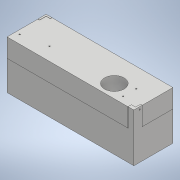
# Autodesk Inventor part: 10руб
Saved by Autodesk Inventor 2020 (Build 240168000, 168)
## iProperties
Created: 2020-02-01
Part Number: 10руб
Material: Типовые
Document SubType Name: Modeling
Designer: Css38
Density: 1 g/cm^3
Appearance: По умолчанию
Author: Css38
Autodesk Inventor part; units mm, degrees
ref_plane "YZ Plane" through (0, 0, 0) normal (1, 0, 0) x (0, 1, 0)
ref_plane "XZ Plane" through (0, 0, 0) normal (0, 1, 0) x (-1, 0, 0)
sketch "Эскиз1" plane through (0, 0, 0) normal (0, 0, 1) x (1, 0, 0)
  line L0 (-76.25, 23.5) -> (76.25, 23.5)
  line L1 (76.25, 23.5) -> (76.25, -23.5)
  line L2 (76.25, -23.5) -> (-76.25, -23.5)
  line L3 (-76.25, -23.5) -> (-76.25, 23.5)
  line L4 (-76.25, 23.5) -> (76.25, -23.5) construction
  line L5 (76.25, 23.5) -> (-76.25, -23.5) construction
  point P0 (0, 0)
  point P1 (0, 0)
  dimension "d35" = 152.5
  dimension "d36" = 47
  constraints: 12 end point, 2 parallel, 1 coincident, 1 horizontal, 1 midpoint, 1 perpendicular
  measures "d35" distance of L1.end L2.end
  measures "d36" distance of L2.end L0.start
extrude "Выдавливание1" add sketch "Эскиз1" along normal blind 30
sketch "Эскиз2" plane through (0, 0, 30) normal (0, 0, 1) x (1, 0, 0)
  line L0 (76.25, 23.5) -> (76.25, -23.5) construction
  line L1 (76.25, -23.5) -> (-76.25, -23.5) construction
  line L2 (-76.25, -23.5) -> (-76.25, 23.5) construction
  line L3 (-76.25, 23.5) -> (76.25, 23.5) construction
  line L4 (74.25, -19.5) -> (50.25, -19.5)
  line L5 (50.25, -19.5) -> (50.25, 4.5)
  line L6 (50.25, 4.5) -> (74.25, 4.5)
  line L7 (74.25, 4.5) -> (74.25, -19.5)
  point P0 (0, 0)
  dimension "d40" = 24
  dimension "d138" = 2
  dimension "d139" = 4
  constraints: 8 end point, 2 parallel, 2 perpendicular, 1 horizontal
  measures "d40" distance of L5.end L6.end
  measures "d138" distance between parallel lines of L0 L7
  measures "d139" distance between parallel lines of L1 L4
extrude "Выдавливание2" cut sketch "Эскиз2" against normal up to next
sketch "Эскиз3" plane through (0, 0, 30) normal (0, 0, 1) x (1, 0, 0)
  line L0 (50.25, 4.5) -> (50.25, -19.5)
  line L1 (50.25, -19.5) -> (74.25, -19.5)
  line L2 (74.25, -19.5) -> (74.25, 4.5)
  line L3 (74.25, 4.5) -> (50.25, 4.5)
  line L4 (76.25, 23.5) -> (76.25, -23.5) construction
  line L5 (76.25, -23.5) -> (-76.25, -23.5) construction
  line L6 (-76.25, 23.5) -> (76.25, 23.5) construction
  line L7 (76.25, 23.5) -> (-76.25, 23.5) projected
  line L8 (-76.25, 23.5) -> (76.25, 23.5)
  line L9 (76.25, 23.5) -> (76.25, -23.5)
  line L10 (76.25, -23.5) -> (-76.25, -23.5)
  line L11 (-76.25, 23.5) -> (-76.25, 21.5)
  line L12 (-76.25, 23.5) -> (-76.25, -23.5) construction
  line L13 (-76.25, 21.5) -> (3.25, 21.5)
  line L14 (3.25, 21.5) -> (3.25, 4.5)
  line L15 (3.25, 4.5) -> (23.25, 4.5)
  line L16 (23.25, 4.5) -> (23.25, -19.5)
  line L17 (23.25, -19.5) -> (-76.25, -19.5)
  line L18 (-76.25, -23.5) -> (-76.25, -19.5)
  line L19 (-76.25, -23.5) -> (76.25, -23.5) projected
  line L20 (76.25, -23.5) -> (76.25, 23.5) projected
  line L21 (74.25, -19.5) -> (50.25, -19.5) projected
  line L22 (50.25, -19.5) -> (50.25, 4.5) projected
  line L23 (50.25, 4.5) -> (74.25, 4.5) projected
  line L24 (74.25, 4.5) -> (74.25, -19.5) projected
  dimension "d50" = 2
  dimension "d52" = 20
  dimension "d63" = 27
  constraints: 34 end point, 13 collinear, 4 perpendicular, 2 parallel, 2 point on line
  measures "d50" distance of L6.start L11.end
  measures "d52" distance between parallel lines of L14 L16
  measures "d63" distance between parallel lines of L0 L16
extrude "Выдавливание4" add sketch "Эскиз3" along normal blind 3
sketch "Эскиз4" plane through (0, 0, 33) normal (0, 0, 1) x (1, 0, 0)
  line L0 (50.25, 4.5) -> (50.25, -19.5) construction
  line L1 (50.25, -19.5) -> (74.25, -19.5) construction
  line L2 (74.25, -19.5) -> (74.25, 4.5) construction
  line L3 (74.25, 4.5) -> (50.25, 4.5) construction
  line L4 (76.25, 23.5) -> (76.25, -23.5) projected
  line L5 (76.25, -23.5) -> (-76.25, -23.5) projected
  line L6 (-76.25, -23.5) -> (-76.25, -19.5) projected
  line L7 (-76.25, -19.5) -> (23.25, -19.5) projected
  line L8 (23.25, -19.5) -> (23.25, 4.5) projected
  line L9 (23.25, 4.5) -> (3.25, 4.5) projected
  line L10 (3.25, 4.5) -> (3.25, 21.5) projected
  line L11 (3.25, 21.5) -> (-76.25, 21.5) projected
  line L12 (-76.25, 21.5) -> (-76.25, 23.5) projected
  line L13 (-76.25, 23.5) -> (76.25, 23.5) projected
  line L14 (23.25, -19.5) -> (23.25, 4.5) projected
  line L15 (23.25, 4.5) -> (50.25, 4.5) construction
  line L16 (50.25, 4.5) -> (50.25, -19.5) projected
  line L17 (50.25, -19.5) -> (23.25, -19.5) construction
  circle A0 centre (36.75, -7.5) radius 11.75
  line L18 (36.75, -7.5) -> (36.75, 4.5) construction
  line L19 (36.75, -7.5) -> (36.75, -19.5) construction
  line L20 (50.25, -19.5) -> (50.25, 4.5) construction
  line L21 (36.75, -7.5) -> (23.25, -7.5) construction
  line L22 (36.75, -7.5) -> (50.25, -7.5) construction
  point P0 (0, 0)
  dimension "d55" = 23.5
  constraints: 12 end point, 4 midpoint, 3 perpendicular, 2 collinear, 1 centre point, 1 point on line, 1 other
  measures "d55" diameter of A0
extrude "Выдавливание7" add sketch "Эскиз4" along normal blind 25
sketch "Эскиз6" plane through (23.25, -19.5, 30) normal (-1, 0, 0) x (0, 0, 1)
  line L0 (3, 0.25) -> (3, 23.75) construction
  line L1 (0, 24) -> (28, 24) projected
  line L2 (0, 0) -> (28, 0) projected
  line L3 (3, 24) -> (5.7, 24)
  line L4 (5.7, 24) -> (5.7, 0)
  line L5 (5.7, 0) -> (3, 0)
  line L6 (3, 0) -> (3, 24)
  point P0 (-30, 19.5)
  dimension "d66" = 2.7
  constraints: 8 end point, 2 parallel, 2 point on line, 1 collinear, 1 horizontal, 1 perpendicular
  measures "d66" distance of L4.end L5.end
extrude "Выдавливание8" cut sketch "Эскиз6" against normal up to surface (51 mm away) from surface at 0
sketch "Эскиз7" plane through (0, 0, 58) normal (0, 0, 1) x (1, 0, 0)
  line L0 (76.25, -23.5) -> (-76.25, -23.5) projected
  line L1 (-76.25, 23.5) -> (76.25, 23.5) projected
  line L2 (76.25, -23.5) -> (-76.25, -23.5)
  line L3 (-76.25, -23.5) -> (-76.25, 23.5)
  line L4 (-76.25, 23.5) -> (76.25, 23.5)
  line L5 (76.25, 23.5) -> (76.25, -23.5)
  circle A0 centre (36.75, -7.5) radius 11.75 projected
  point P0 (0, 0)
  constraints: 8 end point, 2 parallel, 1 horizontal, 1 perpendicular
extrude "Выдавливание9" add sketch "Эскиз7" against normal blind 17.15
ref_plane "РабПлоскость1" through (74.25, -19.5, 35.7) normal (0, 0, -1) x (-1, 0, 0)
split body "Разделение1" result two bodies by plane through (74.25, -19.5, 35.7) normal (0, 0, -1) first body at (-34.0833, 1.5, 0.5)
sketch "Эскиз21" plane through (0, 0, 30) normal (0, 0, 1) x (1, 0, 0)
  line L0 (-76.25, -19.5) -> (23.25, -19.5) construction
  line L1 (23.25, -19.5) -> (23.25, 4.5) construction
  line L2 (23.25, 4.5) -> (3.25, 4.5) construction
  line L3 (3.25, 4.5) -> (3.25, 21.5) construction
  line L4 (3.25, 21.5) -> (-76.25, 21.5) construction
  line L5 (-76.25, -19.5) -> (-76.25, 21.5) construction
  line L6 (-76.25, -23.5) -> (-76.25, -19.5) construction
  line L7 (76.25, -23.5) -> (-76.25, -23.5) construction
  line L8 (76.25, 23.5) -> (76.25, -23.5) construction
  line L9 (74.25, 4.5) -> (50.25, 4.5) construction
  line L10 (50.25, 4.5) -> (50.25, -19.5) construction
  line L11 (50.25, -19.5) -> (74.25, -19.5) construction
  line L12 (74.25, -19.5) -> (74.25, 4.5) construction
  line L13 (-76.25, -19.5) -> (-43.25, -19.5)
  line L14 (-43.25, -19.5) -> (-43.25, -7)
  line L15 (-43.25, -7) -> (-76.25, -7)
  line L16 (-76.25, -7) -> (-76.25, -19.5)
  line L17 (-76.25, 21.5) -> (-76.25, 23.5) projected
  line L18 (-76.25, 23.5) -> (76.25, 23.5) projected
  point P0 (0, 0)
  dimension "d140" = 33
  dimension "d141" = 12.5
  constraints: 8 end point, 2 parallel, 1 horizontal, 1 perpendicular
  measures "d140" distance of L15.end L14.end
  measures "d141" distance of L14.end L13.end
extrude "Выдавливание26" cut sketch "Эскиз21" against normal blind 28 bodies 2
sketch "Эскиз22" plane through (0, 0, 2) normal (0, 0, 1) x (1, 0, 0)
  line L0 (76.25, 23.5) -> (76.25, -23.5) construction
  line L1 (76.25, -23.5) -> (-76.25, -23.5) construction
  line L2 (-76.25, -23.5) -> (-76.25, -19.5) construction
  line L3 (-76.25, -19.5) -> (-76.25, -7) construction
  line L4 (-43.25, -7) -> (-76.25, -7) construction
  line L5 (-43.25, -19.5) -> (-43.25, -7) construction
  line L6 (-76.25, -19.5) -> (-43.25, -19.5) construction
  line L7 (-76.25, -7) -> (-76.25, 23.5) construction
  line L8 (74.25, 4.5) -> (50.25, 4.5) construction
  line L9 (50.25, 4.5) -> (50.25, -19.5) construction
  line L10 (50.25, -19.5) -> (74.25, -19.5) construction
  line L11 (74.25, -19.5) -> (74.25, 4.5) construction
  line L12 (-43.25, -7) -> (-47.75, -7)
  line L13 (-47.75, -7) -> (-47.75, -19.5)
  line L14 (-47.75, -19.5) -> (-43.25, -19.5)
  line L15 (-43.25, -19.5) -> (-43.25, -7)
  line L16 (-76.25, 23.5) -> (76.25, 23.5) projected
  point P0 (0, 0)
  dimension "d144" = 4.5
  constraints: 8 end point, 2 parallel, 1 horizontal, 1 perpendicular, 1 point on line
  measures "d144" distance of L14.end L13.end
extrude "Выдавливание27" add sketch "Эскиз22" along normal blind 18 bodies 2
sketch "Эскиз23" plane through (0, 0, 20) normal (0, 0, 1) x (1, 0, 0)
  line L0 (76.25, 23.5) -> (76.25, -23.5) construction
  line L1 (76.25, -23.5) -> (-76.25, -23.5) construction
  line L2 (-76.25, -23.5) -> (-76.25, -19.5) construction
  line L3 (-76.25, -19.5) -> (-47.75, -19.5) construction
  line L4 (-47.75, -19.5) -> (-47.75, -7) construction
  line L5 (-43.25, -7) -> (-47.75, -7) construction
  line L6 (-43.25, -19.5) -> (-43.25, -7) construction
  line L7 (-47.75, -19.5) -> (-43.25, -19.5) construction
  line L8 (-76.25, -7) -> (-76.25, 23.5) construction
  line L9 (-47.75, -7) -> (-76.25, -7) construction
  line L10 (74.25, 4.5) -> (50.25, 4.5) construction
  line L11 (50.25, 4.5) -> (50.25, -19.5) construction
  line L12 (50.25, -19.5) -> (74.25, -19.5) construction
  line L13 (74.25, -19.5) -> (74.25, 4.5) construction
  line L14 (-47.75, -19.5) -> (-47.75, -7) construction
  line L15 (-43.25, -7) -> (-47.75, -19.5) construction
  line L16 (-47.75, -7) -> (-43.25, -19.5) construction
  circle A0 centre (-45.5, -13.25) radius 0.75
  line L17 (-76.25, 23.5) -> (76.25, 23.5) projected
  point P0 (0, 0)
  dimension "d147" = 1.5
  constraints: 4 end point, 1 centre point, 1 midpoint
  measures "d147" diameter of A0
extrude "Выдавливание28" cut sketch "Эскиз23" against normal blind 3 bodies 2
sketch "Эскиз24" plane through (0, 0, 30) normal (0, 0, 1) x (1, 0, 0)
  line L0 (76.25, 23.5) -> (76.25, -23.5) construction
  line L1 (76.25, -23.5) -> (-76.25, -23.5) construction
  line L2 (-76.25, -23.5) -> (-76.25, -19.5) construction
  line L3 (-76.25, -19.5) -> (-43.25, -19.5) construction
  line L4 (-43.25, -19.5) -> (-43.25, -7) construction
  line L5 (-43.25, -7) -> (-76.25, -7) construction
  line L6 (-76.25, -7) -> (-76.25, 21.5) construction
  line L7 (-43.25, -19.5) -> (23.25, -19.5) construction
  line L8 (23.25, -19.5) -> (23.25, 4.5) construction
  line L9 (23.25, 4.5) -> (3.25, 4.5) construction
  line L10 (3.25, 4.5) -> (3.25, 21.5) construction
  line L11 (3.25, 21.5) -> (-76.25, 21.5) construction
  line L12 (74.25, 4.5) -> (50.25, 4.5) construction
  line L13 (50.25, 4.5) -> (50.25, -19.5) construction
  line L14 (50.25, -19.5) -> (74.25, -19.5) construction
  line L15 (74.25, -19.5) -> (74.25, 4.5) construction
  line L16 (-43.25, -7) -> (-43.25, -19.5) construction
  line L17 (-76.25, -19.5) -> (-76.25, -7) construction
  line L18 (-65.25, -13.25) -> (-46.7028, 16.4317)
  line L19 (-46.7028, 16.4317) -> (-25.4596, -7.5)
  line L20 (-25.4596, -7.5) -> (23.5404, -7.5)
  line L21 (-76.25, 21.5) -> (-76.25, 23.5) projected
  line L22 (-76.25, 23.5) -> (76.25, 23.5) projected
  point P0 (0, 0)
  point P1 (-43.25, -13.25)
  point P2 (-43.25, -13.25)
  point P3 (50.25, -7.5)
  dimension "d150" = 11
  dimension "d151" = 35
  dimension "d152" = 49
  dimension "d154" = 32
  dimension "d155" = 58
  constraints: 6 end point, 3 midpoint, 1 horizontal, 1 horizontal alignment, 1 point on line
  measures "d150" distance from line of L17 L18.start
  measures "d151" distance of L18.start L18.end
  measures "d152" distance of L19.end L20.end
  measures "d154" distance of L18.end L19.end
  measures "d155" angle of L7 L18
sketch "Эскиз20" plane through (0, 0, 58) normal (0, 0, 1) x (1, 0, 0)
  line L0 (-76.25, -23.5) -> (76.25, -23.5) construction
  line L1 (60.5, -23.5) -> (60.5, 8) construction
  line L2 (60.5, 8) -> (50.5, 8) construction
  circle A0 centre (36.75, -7.5) radius 11.75 construction
  line L3 (60.5, -23.5) -> (-46, -23.5) construction
  line L4 (-46, -23.5) -> (-46, 8) construction
  line L5 (-76.25, -23.5) -> (76.25, -23.5) construction
  line L6 (-76.25, 23.5) -> (-76.25, -23.5) construction
  circle A1 centre (-71.25, -13.4) radius 0.5
  line L7 (-36, 8) -> (-36, -23.5) construction
  line L8 (50.5, -23.5) -> (50.5, 8) construction
  line L9 (-36, 8) -> (-46, 8) construction
  line L10 (50.5, 8) -> (-36, 8) construction
  line L11 (-46, 8) -> (-36, -23.5) construction
  line L12 (-36, 8) -> (-46, -23.5) construction
  line L13 (60.5, 8) -> (50.5, -7.75) construction
  line L14 (50.5, -7.75) -> (60.5, -23.5) construction
  line L15 (50.5, -23.5) -> (60.5, -7.75) construction
  line L16 (50.5, 8) -> (60.5, -7.75) construction
  circle A2 centre (-41, -7.75) radius 0.5
  circle A3 centre (55.5, 0.125) radius 0.5
  circle A4 centre (55.5, -15.625) radius 0.5
  point P0 (0, 0)
  dimension "d129" = 31.5
  dimension "d157" = 5
  dimension "d158" = 10.1
  dimension "d159" = 106.5
  dimension "d160" = 2
  dimension "d161" = 10
  dimension "d162" = 1
  constraints: 28 end point, 5 midpoint, 5 perpendicular, 4 centre point, 4 horizontal, 3 equal length, 3 equal radius, 2 point on line, 1 collinear, 1 vertical
  measures "d129" distance of L1.end L1.start
  measures "d157" distance from line of L6 A1.centre
  measures "d158" distance from line of L0 A1.centre
  measures "d159" distance of L1.end L4.end
  measures "d160" distance edge to line of A0 L8
  measures "d161" distance of L1.end L2.end
  measures "d162" diameter of A2
hole "Отверстие1" at (-71.25, -13.4, 58) at (-41, -7.75, 58) at (55.5, 0.125, 58) at (55.5, -15.625, 58) direction (0, 0, -1) diameter 1 depth 4 tip angle 118 countersink diameter 1.5 countersink angle 90 bodies 3
sketch "Эскиз25" plane through (0, 0, 30) normal (0, 0, 1) x (1, 0, 0)
  line L0 (-76.25, -23.5) -> (-76.25, -19.5) construction
  line L1 (-76.25, -19.5) -> (-43.25, -19.5) construction
  line L2 (-43.25, -19.5) -> (-43.25, -7) construction
  line L3 (-43.25, -7) -> (-76.25, -7) construction
  line L4 (-76.25, -7) -> (-76.25, 21.5) construction
  line L5 (-76.25, 21.5) -> (-76.25, 23.5) construction
  line L6 (-76.25, 23.5) -> (76.25, 23.5) construction
  line L7 (76.25, 23.5) -> (76.25, -23.5) construction
  line L8 (76.25, -23.5) -> (-76.25, -23.5) construction
  line L9 (-43.25, -19.5) -> (23.25, -19.5) construction
  line L10 (23.25, -19.5) -> (23.25, 4.5) construction
  line L11 (23.25, 4.5) -> (3.25, 4.5) construction
  line L12 (3.25, 4.5) -> (3.25, 21.5) construction
  line L13 (3.25, 21.5) -> (-76.25, 21.5) construction
  line L14 (74.25, 4.5) -> (50.25, 4.5) construction
  line L15 (50.25, 4.5) -> (50.25, -19.5) construction
  line L16 (50.25, -19.5) -> (74.25, -19.5) construction
  line L17 (74.25, -19.5) -> (74.25, 4.5) construction
  line L18 (-76.25, 23.5) -> (-69.25, 23.5)
  line L19 (-69.25, 23.5) -> (-69.25, 21.5)
  line L20 (-69.25, 21.5) -> (-74.25, 21.5)
  line L21 (-74.25, 21.5) -> (-74.25, 13.5)
  line L22 (-74.25, 13.5) -> (-76.25, 13.5)
  line L23 (-76.25, 13.5) -> (-76.25, 23.5)
  line L24 (76.25, -23.5) -> (69.25, -23.5)
  line L25 (69.25, -23.5) -> (69.25, -19.5)
  line L26 (69.25, -19.5) -> (74.25, -19.5)
  line L27 (74.25, -19.5) -> (74.25, -13.5)
  line L28 (74.25, -13.5) -> (76.25, -13.5)
  line L29 (76.25, -13.5) -> (76.25, -23.5)
  point P0 (0, 0)
  dimension "d170" = 10
  dimension "d171" = 5
  constraints: 24 end point, 9 perpendicular, 3 parallel, 2 horizontal, 1 point on line, 1 vertical
  measures "d170" distance of L5.end L22.end
  measures "d171" distance of L19.end L20.end
extrude "Выдавливание29" add sketch "Эскиз25" along normal blind 28.1 bodies 2
sketch "Эскиз26" plane through (0, 0, 58) normal (0, 0, 1) x (1, 0, 0)
  line L0 (74.25, -13.5) -> (76.25, -13.5) construction
  line L1 (76.25, -13.5) -> (76.25, -23.5) construction
  line L2 (76.25, -23.5) -> (69.25, -23.5) construction
  line L3 (69.25, -23.5) -> (69.25, -19.5) construction
  line L4 (69.25, -19.5) -> (74.25, -19.5) construction
  line L5 (74.25, -19.5) -> (74.25, -13.5) construction
  line L6 (-74.25, 21.5) -> (-74.25, 13.5) construction
  line L7 (-74.25, 13.5) -> (-76.25, 13.5) construction
  line L8 (-76.25, 13.5) -> (-76.25, 23.5) construction
  line L9 (-76.25, 23.5) -> (-69.25, 23.5) construction
  line L10 (-69.25, 23.5) -> (-69.25, 21.5) construction
  line L11 (-69.25, 21.5) -> (-74.25, 21.5) construction
  circle A0 centre (55.5, 0.125) radius 0.75 construction
  circle A1 centre (-71.25, -13.4) radius 0.75 construction
  circle A2 centre (-41, -7.75) radius 0.75 construction
  circle A3 centre (55.5, -15.625) radius 0.75 construction
  line L12 (-76.25, -23.5) -> (-76.25, 23.5) construction
  line L13 (-76.25, 23.5) -> (76.25, 23.5) construction
  line L14 (76.25, 23.5) -> (76.25, -23.5) construction
  line L15 (76.25, -23.5) -> (-76.25, -23.5) construction
  circle A4 centre (36.75, -7.5) radius 11.75 construction
  line L16 (-74.15, 13.4) -> (-74.15, 21.4)
  line L17 (-74.15, 21.4) -> (-69.15, 21.4)
  line L18 (-69.15, 21.4) -> (-69.15, 23.6)
  line L19 (-69.15, 23.6) -> (-76.35, 23.6)
  line L20 (-76.35, 23.6) -> (-76.35, 13.4)
  line L21 (-76.35, 13.4) -> (-74.15, 13.4)
  line L22 (74.15, -19.4) -> (69.15, -19.4)
  line L23 (69.15, -19.4) -> (69.15, -23.6)
  line L24 (69.15, -23.6) -> (76.35, -23.6)
  line L25 (76.35, -23.6) -> (76.35, -13.4)
  line L26 (76.35, -13.4) -> (74.15, -13.4)
  line L27 (74.15, -13.4) -> (74.15, -19.4)
  point P0 (0, 0)
  dimension "d174" = 0.1
  dimension "d175" = 0.1
  constraints: 24 end point, 10 other
  measures "d174" distance between parallel lines of L6 L16
  measures "d175" distance between parallel lines of L4 L22
extrude "Выдавливание30" cut sketch "Эскиз26" against normal through all bodies 3
sketch "Эскиз27" plane through (76.25, -23.5, 0) normal (1, 0, 0) x (0, 0, -1)
  line L0 (0, 4) -> (-58.1, 4) construction
  line L1 (-58.1, 4) -> (-52.1, 10) construction
  line L2 (-35.7, 10) -> (-58.1, 10) construction
  line L3 (-58.1, 0) -> (-58.1, 10) construction
  line L4 (-58.1, 10) -> (-52.1, 4) construction
  circle A0 centre (-55.1, 7) radius 0.5
  point P0 (0, 23.5)
  dimension "d178" = 1
  constraints: 4 end point, 2 perpendicular, 2 point on line, 1 centre point, 1 midpoint
  measures "d178" diameter of A0
hole "Отверстие2" at (76.25, -16.5, 55.1) direction (-1, 0, 0) diameter 1 end through all countersink diameter 1.5 countersink angle 90 bodies 2
sketch "Эскиз28" plane through (-76.25, -23.5, 0) normal (-1, 0, 0) x (0, 0, 1)
  circle A0 centre (55.1, 7) radius 0.5 construction
  line L0 (58.1, 45) -> (30, 45) construction
  line L1 (35.7, 45) -> (58.1, 45) construction
  line L2 (58.1, 45) -> (50.1, 37) construction
  line L3 (30, 37) -> (58.1, 37) construction
  line L4 (58.1, 37) -> (50.1, 45) construction
  circle A1 centre (54.1, 41) radius 0.5
  point P0 (0, 23.5)
  constraints: 4 end point, 2 perpendicular, 2 point on line, 1 centre point, 1 equal radius, 1 midpoint
hole "Отверстие3" at (-76.25, 17.5, 54.1) direction (1, 0, 0) diameter 1 end through all countersink diameter 1.5 countersink angle 90 bodies 2
sketch "Эскиз29" plane through (74.15, -19.4, 58) normal (1, 0, 0) x (0, 0, -1)
  circle A0 centre (2.9, 2.9) radius 0.5 construction
  circle A1 centre (3, 2.9) radius 0.5
  point P0 (58, 19.4)
  dimension "d193" = 0.1
  constraints: 1 centre point, 1 equal radius, 1 horizontal alignment
  measures "d193" distance of A0.centre A1.centre
hole "Отверстие4" at (74.15, -16.5, 55) direction (-1, 0, 0) diameter 1 depth 3 tip angle 118 countersink diameter 1.5 countersink angle 90 bodies 3
sketch "Эскиз30" plane through (-74.15, 13.4, 58) normal (-1, 0, 0) x (0, 0, 1)
  circle A0 centre (-3, -29.9) radius 0.5 construction
  line L0 (0, 8) -> (0, 0) construction
  circle A1 centre (-3, 4) radius 0.5
  point P0 (-58, -13.4)
  point P1 (0, 4)
  constraints: 1 centre point, 1 equal radius, 1 horizontal alignment, 1 midpoint, 1 vertical alignment
hole "Отверстие5" at (-74.15, 17.4, 55) direction (1, 0, 0) diameter 1 depth 3 tip angle 118 countersink diameter 1.5 countersink angle 90 bodies 3
